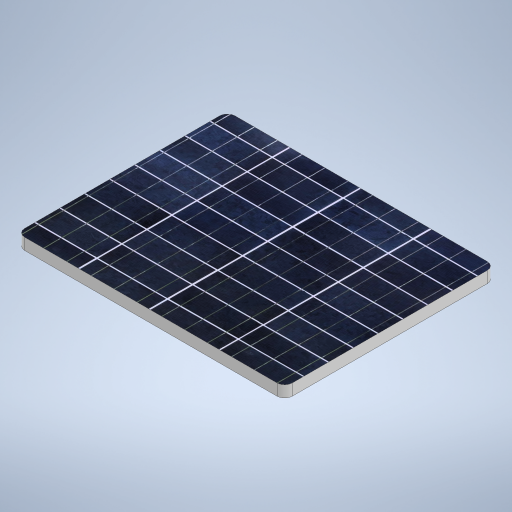
# Autodesk Inventor part: solar-panel
Saved by Autodesk Inventor 2023 (Build 270158000, 158)
## iProperties
Created: 2023-01-30
Part Number: solar-panel
Material: Generic
Document SubType Name: Modeling
Designer: ringl
Density: 1 g/cm^3
Appearance: Default
Author: ringl
Autodesk Inventor part; units mm, degrees
ref_plane "YZ Plane" through (0, 0, 0) normal (1, 0, 0) x (0, 1, 0)
ref_plane "XZ Plane" through (0, 0, 0) normal (0, 1, 0) x (-1, 0, 0)
ref_plane "XY Plane" through (0, 0, 0) normal (0, 0, 1) x (1, 0, 0)
sketch "Sketch1" plane through (0, 0, 0) normal (0, 1, 0) x (-1, 0, 0)
  line L0 (0, 0) -> (70, 0)
  line L1 (70, 0) -> (70, -55)
  line L2 (70, -55) -> (0, -55)
  line L3 (0, -55) -> (0, 0)
  dimension "d0" = 70
  dimension "d1" = 55
  constraints: 8 end point, 2 parallel, 1 horizontal, 1 perpendicular
  measures "d0" distance of L1.end L2.end
  measures "d1" distance of L0.end L1.end
extrude "Extrusion1" add sketch "Sketch1" along normal blind 3
fillet "Fillet1" radius 2 4 edges at (-70, 1.5, 0) (0, 1.5, 0) (0, 1.5, -55) (-70, 1.5, -55)
sketch "Sketch2" plane through (0, 3, 0) normal (0, 1, 0) x (1, 0, 0)
  line L0 (-80, 71.1328) -> (10, 71.1328) construction
  line L1 (10, 71.1328) -> (10, -15) construction
  line L2 (10, -15) -> (-80, -15) construction
  line L3 (-80, -15) -> (-80, 71.1328) construction
  point P0 (0, 0)
  dimension "d20" = 10
  dimension "d21" = 15
  dimension "d31" = 90
  constraints: 2 other
  measures "d20" distance from line of point (0, 0) L1
  measures "d21" distance from line of point (0, 0) L2
  measures "d31" distance of L0.start L0.end
decal "Decal1"
body "Solid1"
